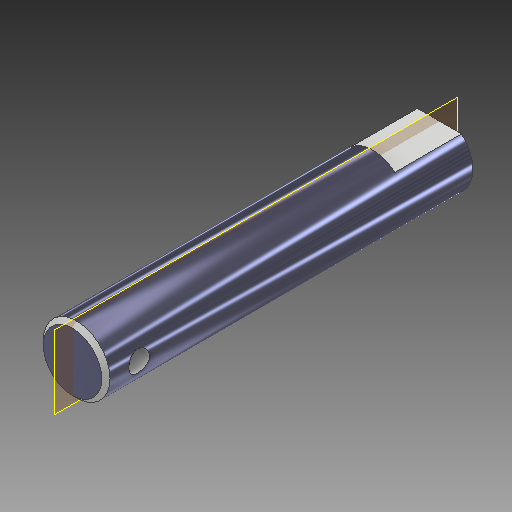
# Autodesk Inventor part: reverse gear crankshaft outer rod
Saved by Autodesk Inventor 2017 (Build 210142000, 142)
## iProperties
Created: 2018-10-30
Part Number: reverse gear crankshaft outer rod
Material: Generic
Document SubType Name: Modeling
Designer: User
Density: 1 g/cm^3
Appearance: Default
Author: User
Autodesk Inventor part; units mm, degrees
ref_plane "XZ Plane" through (0, 0, 0) normal (0, 1, 0) x (-1, 0, 0)
ref_plane "XY Plane" through (0, 0, 0) normal (0, 0, 1) x (1, 0, 0)
sketch "Sketch2" plane through (0, 0, 0) normal (0, 1, 0) x (-1, 0, 0)
  circle A0 centre (0, 0) radius 4
  dimension "d9" = 8
  constraints: 1 centre point, 1 coincident
  measures "d9" diameter of A0
extrude "Extrusion1" add sketch "Sketch2" along normal blind 44
chamfer "Chamfer1" distance 0.5 angle 45 1 edges at (4, 0, 0)
sketch "Sketch3" plane through (0, 44, 0) normal (0, 1, 0) x (1, 0, 0)
  line L0 (0, 0) -> (0, -3) construction
  line L1 (0, -3) -> (-4, -3)
  line L2 (0, -3) -> (4, -3)
  line L3 (4, -3) -> (4, -6)
  line L4 (4, -6) -> (-4, -6)
  line L5 (-4, -6) -> (-4, -3)
  dimension "d15" = 3
  dimension "d16" = 4
  dimension "d17" = 4
  dimension "d18" = 3
  constraints: 12 end point, 2 horizontal, 2 perpendicular, 2 vertical
  measures "d15" distance of L0.start L0.end
  measures "d16" distance of L0.end L1.end
  measures "d17" distance of L0.end L2.end
  measures "d18" distance of L2.end L3.end
extrude "Extrusion2" cut sketch "Sketch3" against normal blind 8
ref_plane "Work Plane1" through (-4, 0, 0) normal (1, 0, 0) x (0, 1, 0)
sketch "Sketch4" plane through (-4, 0, 0) normal (1, 0, 0) x (0, 1, 0)
  line L0 (0.5, 4) -> (0.5, -4) construction
  line L1 (0.5, 0) -> (4, 0) construction
  circle A0 centre (4, 0) radius 1.25
  point P0 (0, 0)
  dimension "d23" = 2.5
  dimension "d24" = 3.5
  constraints: 2 end point, 1 centre point, 1 coincident, 1 horizontal, 1 midpoint
  measures "d23" diameter of A0
  measures "d24" distance of L1.start A0.centre
extrude "Extrusion3" cut sketch "Sketch4" along normal through all
body "Solid1"
